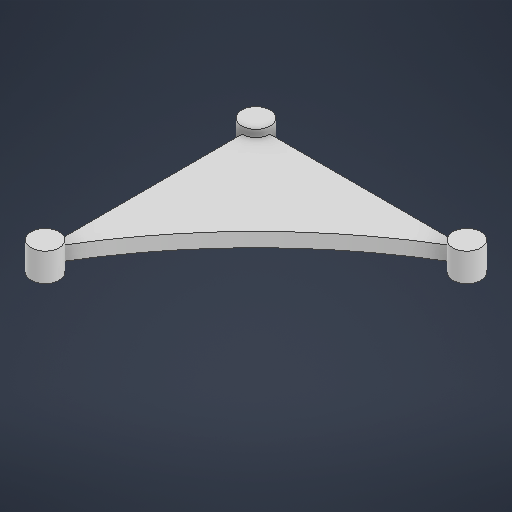
# Autodesk Inventor part: Knee
Saved by Autodesk Inventor 2027 (Build 310192060, 192F)
## iProperties
Created: 2026-08-01
Part Number: Knee
Material: Ogólny
Document SubType Name: Modeling
Designer: User
Density: 1 g/cm^3
Appearance: Domyślna
Author: User
Autodesk Inventor part; units mm, degrees
ref_plane "YZ Plane" through (0, 0, 0) normal (1, 0, 0) x (0, 1, 0)
ref_plane "XZ Plane" through (0, 0, 0) normal (0, 1, 0) x (-1, 0, 0)
ref_plane "XY Plane" through (0, 0, 0) normal (0, 0, 1) x (1, 0, 0)
sketch "Szkic1" plane through (0, 0, 0) normal (0, 1, 0) x (-1, 0, 0)
  line L0 (0, 0) -> (0, -15)
  circle A0 centre (0, 0) radius 1
  circle A1 centre (0, -15) radius 1
  line L1 (0, -15) -> (-15, -15)
  line L2 (0, -15) -> (15, -15) construction
  circle A2 centre (-15, -15) radius 1
  arc A3 (-15, -15) -> (0, 0) centre (-34.7718, 19.7718) ccw
  point P0 (-14.137, -14.4949)
  point P1 (-14, -15)
  point P2 (-1, -15)
  point P3 (0, -14)
  point P4 (0, -1)
  point P5 (-0.5051, -0.863)
  dimension "d0" = 15
  dimension "d1" = 2
  dimension "d2" = 2
  dimension "d3" = 15
  dimension "d4" = 180
  dimension "d5" = 2
  dimension "d6" = 40
  constraints: 6 end point, 4 centre point, 3 coincident, 2 point on circle, 1 collinear, 1 horizontal, 1 vertical
  measures "d0" distance of L0.start L0.end
  measures "d1" diameter of A0
  measures "d2" diameter of A1
  measures "d3" distance of L1.start L1.end
  measures "d4" angle of L2 L1
  measures "d5" diameter of A2
  measures "d6" radius of A3
extrude "Wyciągnięcie proste1" add sketch "Szkic1" along normal mid plane 1
extrude "Wyciągnięcie proste2" add sketch "Szkic1" along normal mid plane 2 contours A3 A0 L0 | L0 A0 A3 | A1 L1 L0 | L0 L1 A1 | A3 L1 A2 | A2 L1 A3
